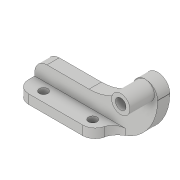
# Autodesk Inventor part: supporty2
Saved by Autodesk Inventor 2018 (Build 220112000, 112)
## iProperties
Created: 2017-12-20
Part Number: supporty2
Material: Generic
Document SubType Name: Modeling
Designer: dsayers
Density: 1 g/cm^3
Appearance: Default
Author: dsayers
Autodesk Inventor part; units mm, degrees
ref_plane "YZ Plane" through (0, 0, 0) normal (1, 0, 0) x (0, 1, 0)
ref_plane "XZ Plane" through (0, 0, 0) normal (0, 1, 0) x (-1, 0, 0)
sketch "Sketch1" plane through (0, 0, 0) normal (0, 0, 1) x (1, 0, 0)
  line L0 (0, 0) -> (63.5, 0)
  line L1 (63.5, 0) -> (63.5, 12.9255)
  line L2 (63.5, 12.9255) -> (0, 12.9255)
  line L3 (0, 12.9255) -> (0, 0)
  line L4 (63.5, 12.9255) -> (50.8, 12.9255)
  line L5 (50.8, 12.9255) -> (50.8, -19.0013)
  line L6 (50.8, -19.0013) -> (63.5, -19.0013)
  line L7 (63.5, -19.0013) -> (63.5, 12.9255)
  point P0 (57.15, -14.2271)
  point P1 (34.4424, 12.9255)
  point P2 (9.0424, 12.9255)
  dimension "d0" = 63.5
  dimension "d2" = 22.7076
  dimension "d3" = 25.4
  dimension "d4" = 27.1526
  dimension "d5" = 0
  dimension "d6" = 6.35
  dimension "d7" = 6.35
  constraints: 16 end point, 4 parallel, 2 horizontal, 2 perpendicular
  measures "d0" distance between parallel lines of L1 L3
  measures "d2" horizontal distance of point (57.15, -14.227) point (34.442, 12.926)
  measures "d3" distance of point (9.042, 12.926) point (34.442, 12.926)
  measures "d4" vertical distance of point (34.442, 12.926) point (57.15, -14.227)
  measures "d5" distance from line of point (34.442, 12.926) L2
  measures "d6" distance from line of point (57.15, -14.227) L1
  measures "d7" distance from line of point (57.15, -14.227) L5
extrude "Extrusion1" add sketch "Sketch1" along normal blind 6.35
sketch "Sketch2" plane through (0, 0, 6.35) normal (0, 0, 1) x (1, 0, 0)
  line L0 (63.5, -19.0013) -> (63.5, 12.9255) projected
  line L1 (50.8, 0) -> (50.8, -19.0013) projected
  line L2 (63.5, 12.9255) -> (0, 12.9255) projected
  point P0 (0, 0)
  point P1 (57.15, -14.2271)
  dimension "d10" = 6.35
  dimension "d11" = 6.35
  dimension "d12" = 27.1526
  measures "d10" distance from line of L0 point (57.15, -14.227)
  measures "d11" distance from line of L1 point (57.15, -14.227)
  measures "d12" distance from line of L2 point (57.15, -14.227)
hole "Hole1" at (57.15, -14.2271, 6.35) direction (0, 0, -1) diameter 5.5 depth 25.4 tip angle 118
sketch "Sketch3" plane through (0, 0, 6.35) normal (0, 0, 1) x (1, 0, 0)
  circle A0 centre (57.15, -14.2271) radius 2.75 projected
  circle A1 centre (57.15, -14.2271) radius 4.7742
  line L0 (50.8, -19.0013) -> (63.5, -19.0013) projected
  point P0 (0, 0)
  constraints: 1 centre point, 1 coincident, 1 tangent
extrude "Extrusion2" add sketch "Sketch3" along normal blind 12.7
fillet "Fillet1" radius 6.35 2 edges at (63.5, -19.0013, 3.175) (50.8, -19.0013, 3.175)
fillet "Fillet2" radius 25.4 2 edges at (50.8, 0, 3.175) (63.5, 12.9255, 3.175)
sketch "Sketch4" plane through (0, 0, 6.35) normal (0, 0, 1) x (1, 0, 0)
  line L0 (0, 12.9255) -> (0, 0) projected
  line L1 (0, 12.9255) -> (40.7924, 12.9255)
  line L2 (40.7924, 12.9255) -> (40.7924, 8.163)
  line L3 (40.7924, 8.163) -> (0, 8.163)
  line L4 (0, 8.163) -> (0, 12.9255)
  circle A0 centre (57.15, -14.2271) radius 2.75 projected
  dimension "d24" = 16.3576
  dimension "d25" = 4.7625
  constraints: 8 end point, 2 parallel, 1 horizontal, 1 perpendicular
  measures "d24" distance from line of A0.centre L2
  measures "d25" distance between parallel lines of L1 L3
extrude "Extrusion3" add sketch "Sketch4" along normal blind 9.525 contours L1 L2 L3 L0
fillet "Fillet3" radius 6.35 2 edges at (40.7924, 10.5443, 15.875) (0, 10.5443, 15.875)
fillet "Fillet4" radius 6.35 1 edges at (40.7924, 10.4727, 6.35)
sketch "Sketch5" plane through (6.35, 8.163, 15.875) normal (0, -1, 0) x (1, 0, 0)
  line L0 (48.05, 3.175) -> (53.55, 3.175) projected
  point P0 (-6.35, -15.875)
  point P1 (2.6924, -5.0739)
  point P2 (28.0924, -5.0739)
  point P3 (50.8, 3.175)
  dimension "d30" = 25.4
  dimension "d31" = 22.7076
  constraints: 1 midpoint
  measures "d30" distance of point (2.692, -5.074) point (28.092, -5.074)
  measures "d31" horizontal distance of point (28.092, -5.074) point (50.8, 3.175)
hole "Hole2" at (9.0424, 8.163, 10.8011) at (34.4424, 8.163, 10.8011) at (57.15, 8.163, 19.05) direction (0, 1, 0) diameter 4.4958 depth 25.4 tip angle 118 clearance for "Flat Head Machine Screw (82)" size "#8" standard "Ansi Unified Screw Threads"
fillet "Fillet5" radius 6.35 1 edges at (0, 0, 3.175)
ref_plane "Work Plane1" through (0, 38.3255, 0) normal (0, 1, 0) x (1, 0, 0)
mirror "Mirror1" about plane through (0, 38.3255, 0) normal (0, 1, 0) of "Extrusion3", "Fillet4", "Fillet5", "Hole2", "Fillet3", "Fillet2", "Fillet1", "Extrusion2", "Hole1", "Extrusion1"
sketch "Sketch6" plane through (0, 12.9255, 0) normal (0, 1, 0) x (1, 0, 0)
  line L0 (75.6078, -32.1869) -> (-9.353, -32.1869)
  line L1 (-9.353, -32.1869) -> (-9.353, 6.0612)
  line L2 (-9.353, 6.0612) -> (75.6078, 6.0612)
  line L3 (75.6078, 6.0612) -> (75.6078, -32.1869)
  point P0 (0, 0)
  constraints: 8 end point, 2 parallel, 1 horizontal, 1 perpendicular
extrude "Extrusion4" cut sketch "Sketch6" against normal blind 101.6
body "Solid1"
